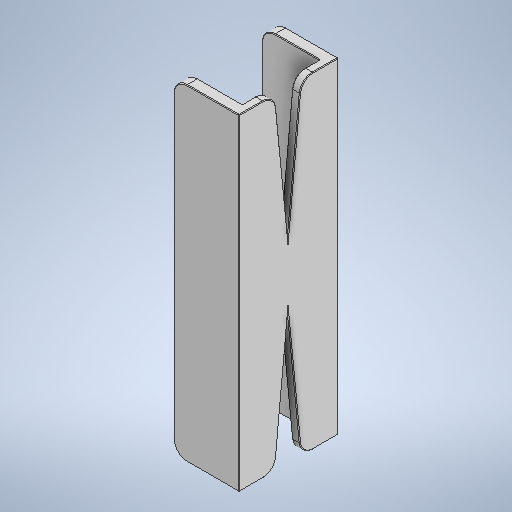
# Autodesk Inventor part: Соединитель
Saved by Autodesk Inventor 2025 (Build 290162000, 162)
## iProperties
Created: 2025-05-20
Part Number: Соединитель
Material: Типовые
Document SubType Name: Modeling
Designer: vinogradov
Density: 1 g/cm^3
Appearance: По умолчанию
Author: vinogradov
Autodesk Inventor part; units mm, degrees
ref_plane "YZ Plane" through (0, 0, 0) normal (1, 0, 0) x (0, 1, 0)
ref_plane "XZ Plane" through (0, 0, 0) normal (0, 1, 0) x (-1, 0, 0)
ref_plane "XY Plane" through (0, 0, 0) normal (0, 0, 1) x (1, 0, 0)
sketch "Эскиз2" plane through (0, 0, 0) normal (0, 1, 0) x (-1, 0, 0)
  line L0 (0, 0) -> (10, 0)
  line L1 (10, 0) -> (10, -1.7)
  line L2 (10, -1.7) -> (1.2, -1.7)
  line L3 (1.2, -1.7) -> (1.2, -13.5)
  line L4 (1.2, -13.5) -> (10, -13.5)
  line L5 (10, -13.5) -> (10, -15.2)
  line L6 (10, -15.2) -> (0, -15.2)
  line L7 (0, -15.2) -> (0, 0)
  dimension "d0" = 10
  dimension "d1" = 1.7
  dimension "d4" = 1.7
  dimension "d5" = 1.2
  dimension "d10" = 15.2
  constraints: 16 end point, 6 perpendicular, 2 point on line, 1 horizontal
  measures "d0" distance of L0.start L0.end
  measures "d1" distance of L0.end L1.end
  measures "d4" distance of L4.end L5.end
  measures "d5" distance between parallel lines of L7 L3
  measures "d10" distance between parallel lines of L6 L0
extrude "Выдавливание1" add sketch "Эскиз2" along normal blind 50
fillet "Сопряжение1" radius 2 4 edges at (-10, 50, -14.35) (-10, 50, -0.85) (-10, 0, -14.35) (-10, 0, -0.85)
sketch "Эскиз3" plane through (0, 0, 0) normal (1, 0, 0) x (0, 0, -1)
  line L0 (13.5, 0) -> (1.7, 0) projected
  line L1 (5.5, 0) -> (7.5, 20)
  line L2 (7.5, 20) -> (9.5, 0)
  line L3 (9.5, 0) -> (5.5, 0)
  line L4 (13.5, 50) -> (1.7, 50) projected
  line L5 (5.5, 50) -> (7.5, 30)
  line L6 (7.5, 30) -> (9.5, 50)
  line L7 (9.5, 50) -> (5.5, 50)
  line L8 (0, 0) -> (0, 50) projected
  point P0 (7.6, 50)
  point P1 (7.5, 0)
  point P2 (7.5, 50)
  point P3 (9.5, 0)
  dimension "d11" = 20
  dimension "d12" = 20
  dimension "d15" = 0
  dimension "d16" = 0
  dimension "d17" = 7.5
  dimension "d18" = 7.5
  dimension "d19" = 4
  dimension "d20" = 4
  constraints: 12 end point, 3 midpoint, 2 horizontal, 2 point on line
  measures "d11" vertical distance of point (7.6, 50) L5.end
  measures "d12" distance from line of L0 L1.end
  measures "d15" horizontal distance of L1.end point (7.5, 0)
  measures "d16" horizontal distance of point (7.5, 50) L5.end
  measures "d17" distance from line of L8 L1.end
  measures "d18" distance from line of L8 L5.end
  measures "d19" distance of L2.end L1.start
  measures "d20" distance of L6.end L5.start
extrude "Выдавливание2" cut sketch "Эскиз3" against normal blind 10
fillet "Сопряжение3" radius 2 4 edges at (-0.6, 0, -9.5) (-0.6, 0, -5.5) (-0.6, 50, -5.5) (-0.6, 50, -9.5)
fillet "Сопряжение4" radius 0.1 47 edges at (-9.4142, 49.4142, -15.2) (-4, 50, -15.2) (-9.4142, 0.5858, -15.2) (-4, 0, -15.2) (-10, 25, -15.2) (-9.4142, 49.4142, -13.5) (-4.6, 50, -13.5) (-9.4142, 0.5858, -13.5) (-4.6, 0, -13.5) (-10, 25, -13.5) (-1.2, 25, -13.5) (-1.2, 49.4829, -9.968) (-1.2, 50, -12.405) (-1.2, 39.0995, -8.41) (-1.2, 49.4829, -5.032) (-1.2, 50, -2.695) (-1.2, 39.0995, -6.59) (0, 49.4829, -5.032) (0, 50, -1.845) (0, 39.0995, -6.59) (0, 49.4829, -9.968) (0, 50, -13.255) (0, 39.0995, -8.41) (-1.2, 0.5171, -9.968) (-1.2, 0, -12.405) (-1.2, 10.9005, -8.41) (0, 0.5171, -9.968) (0, 0, -13.255) (0, 10.9005, -8.41) (-1.2, 0.5171, -5.032) (-1.2, 0, -2.695) (-1.2, 10.9005, -6.59) (0, 0.5171, -5.032) (0, 0, -1.845) (0, 10.9005, -6.59) (-9.4142, 49.4142, -1.7) (-4.6, 50, -1.7) (-9.4142, 0.5858, -1.7) (-4.6, 0, -1.7) (-10, 25, -1.7) (-9.4142, 49.4142, 0) (-4, 50, 0) (-9.4142, 0.5858, 0) (-4, 0, 0) (-10, 25, 0) (0, 25, 0) (0, 25, -15.2)
